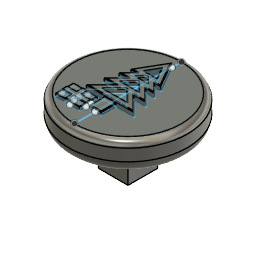
PIN6 (Autodesk Fusion 360 design; units mm, degrees)
Autodesk Fusion 360 part; units mm, degrees
sketch "Sketch1" plane through (0, 0, 0) normal (0, 1, 0) x (1, 0, 0)
  line L0 (0, 0) -> (5, 0)
  line L1 (5, 0) -> (5, 5)
  line L2 (5, 5) -> (0, 5)
  line L3 (0, 5) -> (0, 0)
  dimension "d1" = 5
  dimension "d2" = 5
  constraint horizontal L0
  constraint vertical L1
  constraint horizontal L2
  constraint vertical L3
  constraint coincident L0.start L3.end
  measures "d1" distance of L0.start L0.end
  measures "d2" distance of L0.start L2.end
extrude "Extrude1" add sketch "Sketch1" along normal blind 6
sketch "Sketch2" plane through (0, 6, 0) normal (0, 1, 0) x (-1, 0, 0)
  line L0 (0, -5) -> (0, 0)
  line L1 (0, 0) -> (-5, 0)
  line L2 (-5, 0) -> (-5, -5)
  line L3 (-5, -5) -> (0, -5)
  circle A0 centre (-2.5, -2.5) radius 10
  dimension "d5" = 20
  measures "d5" diameter of A0
extrude "Extrude2" add sketch "Sketch2" along normal blind 5 contours L0 L1 L2 L3 | A0
fillet "Fillet1" radius 2 1 edges at (11.8233, 6, -6.1162)
fillet "Fillet1" radius 1 1 edges at (11.8233, 11, -6.1162)
sketch "Sketch3" plane through (0, 11, 0) normal (0, 1, 0) x (-1, 0, 0)
  circle A0 centre (-2.5, -2.5) radius 9
  line L0 (-2.5, 6.5) -> (-2.5, -11.5)
  line L1 (-2.5, 3) -> (-3.5, 3)
  line L2 (-3.5, 3) -> (-3.5, 0.5)
  line L3 (-3.5, 0.5) -> (-6.5, 0.5)
  line L4 (-6.5, 0.5) -> (-4, -2)
  line L5 (-4, -2) -> (-6, -2)
  line L6 (-6, -2) -> (-4, -4)
  line L7 (-4, -4) -> (-5.5, -4)
  line L8 (-5.5, -4) -> (-4, -5.5)
  line L9 (-4, -5.5) -> (-5, -5.5)
  line L10 (-5, -5.5) -> (-2.5, -9.8301)
  line L11 (0.5, -4) -> (-1, -5.5)
  line L12 (-1, -2) -> (1, -2)
  line L13 (-1, -4) -> (0.5, -4)
  line L14 (-1.5, 0.5) -> (1.5, 0.5)
  line L15 (-2.5, 3) -> (-1.5, 3)
  line L16 (-1.5, 3) -> (-1.5, 0.5)
  line L17 (1.5, 0.5) -> (-1, -2)
  line L18 (0, -5.5) -> (-2.5, -9.8301)
  line L19 (1, -2) -> (-1, -4)
  line L20 (-1, -5.5) -> (0, -5.5)
  line L21 (-1.5, 0.5) -> (-3.5, 0.5)
  line L22 (-4.4238, -0.36) -> (-2.5, -2.2838)
  line L23 (-3.5, -0.36) -> (-4.4238, -0.36)
  line L24 (-1.5, -0.36) -> (-3.5, -0.36)
  line L25 (-1.5, -0.36) -> (-0.5762, -0.36)
  line L26 (-0.5762, -0.36) -> (-2.5, -2.2838)
  line L27 (-3.9238, -2.86) -> (-2.5, -4.2838)
  line L28 (-3.0762, -2.86) -> (-3.9238, -2.86)
  line L29 (-1.9238, -2.86) -> (-3.0762, -2.86)
  line L30 (-1.9238, -2.86) -> (-1.0762, -2.86)
  line L31 (-1.0762, -2.86) -> (-2.5, -4.2838)
  line L32 (-3.4238, -4.86) -> (-2.5, -5.7838)
  line L33 (-3.0762, -4.86) -> (-3.4238, -4.86)
  line L34 (-1.9238, -4.86) -> (-3.0762, -4.86)
  line L35 (-1.9238, -4.86) -> (-1.5762, -4.86)
  line L36 (-1.5762, -4.86) -> (-2.5, -5.7838)
  line L37 (-1.4896, -6.36) -> (-2.5, -8.1101)
  line L38 (-3.5104, -6.36) -> (-2.5, -8.1101)
  line L39 (-3.0762, -6.36) -> (-3.5104, -6.36)
  line L40 (-1.9238, -6.36) -> (-3.0762, -6.36)
  line L41 (-1.9238, -6.36) -> (-1.4896, -6.36)
  line L42 (3.0533, 1.123) -> (-0.9467, 1.123)
  line L43 (-0.9467, 1.123) -> (-0.9467, 4.123)
  line L44 (-0.9467, 4.123) -> (3.0533, 4.123)
  line L45 (3.0533, 4.123) -> (3.0533, 1.123)
  line L46 (1.4833, 4.123) -> (1.4833, 1.123)
  line L47 (1.0533, 4.123) -> (1.0533, 1.123)
  line L48 (1.0533, 2.623) -> (3.0533, 2.623)
  line L49 (3.0533, 2.193) -> (1.0533, 2.193)
  line L50 (3.0533, 3.053) -> (1.0533, 3.053)
  line L51 (0.6233, 4.123) -> (0.6233, 1.123)
  line L52 (-0.9467, 3.053) -> (1.0533, 3.053)
  line L53 (-0.9467, 2.193) -> (1.0533, 2.193)
  dimension "d12" = 60
  dimension "d19" = 0.86
  dimension "d28" = 4
  dimension "d29" = 3
  dimension "d30" = 0.43
  dimension "d31" = 0.43
  dimension "d36" = 2.5
  constraint coincident A0 L0.start
  constraint coincident A0 L0.end
  constraint vertical L0
  constraint coincident L0 L1.start
  constraint perpendicular L0 L1
  constraint perpendicular L1 L2
  constraint perpendicular L2 L3
  constraint perpendicular L2 L5
  constraint parallel L4 L6
  constraint parallel L4 L8
  constraint parallel L3 L9
  constraint coincident L0 L10.end
  constraint symmetric L0 L1.start L15.start
  constraint symmetric L0 L1.end L15.end
  constraint symmetric L0 L2.end L14.start
  constraint symmetric L0 L3.end L14.end
  constraint symmetric L0 L4.end L12.start
  constraint symmetric L0 L5.end L12.end
  constraint symmetric L0 L6.end L13.start
  constraint symmetric L0 L7.end L11.start
  constraint symmetric L0 L8.end L11.end
  constraint symmetric L0 L9.end L18.start
  constraint symmetric L0 L10.end L18.end
  constraint horizontal L42
  constraint vertical L43
  constraint horizontal L44
  constraint vertical L45
  constraint coincident L44 L46.start
  constraint coincident L42 L46.end
  constraint perpendicular L42 L46
  constraint midpoint L44 L47.start
  constraint midpoint L42 L47.end
  constraint midpoint L47 L48.start
  constraint midpoint L45 L48.end
  constraint coincident L45 L49.start
  constraint coincident L47 L49.end
  constraint perpendicular L47 L49
  constraint symmetric L48 L49.start L50.start
  constraint symmetric L48 L49.end L50.end
  constraint symmetric L46.start L47 L51.start
  constraint symmetric L46.end L47 L51.end
  constraint symmetric L47 L49.start L53.start
  constraint symmetric L47 L49.end L53.end
  constraint symmetric L47 L50.start L52.start
  constraint symmetric L47 L50.end L52.end
  measures "d12" angle of L9 L10
  measures "d28" distance of L42.start L42.end
  measures "d29" distance of L42.start L44.end
  measures "d30" distance of L46 L47
  measures "d31" distance of L48 L49
  measures "d36" distance of L1.end L2.end
extrude "Extrude5" add sketch "Sketch3" along normal blind 0.75 contours L0 L3 L4 L5 L6 L7 L8 L9 L10 L21 L22 L23 L24 L27 L28 L29 L32 L33 L34 L38 L39 L40 | L0 L11 L12 L13 L14 L17 L18 L19 L20 L21 L24 L25 L26 L29 L30 L31 L34 L35 L36 L37 L40 L41
extrude "Extrude6" add sketch "Sketch3" along normal blind 0.5 contours L0 L15 L16 L21 | L0 L1 L2 L21
fillet "Fillet2" radius 0.1 27 edges at (2.5, 11.75, -6.36) (3.0052, 11.75, -7.2351) (1.9948, 11.75, -7.2351) (1.25, 11.75, -7.6651) (0.5, 11.75, -5.5) (0.25, 11.75, -4.75) (0.25, 11.75, -4) (0, 11.75, -3) (0, 11.75, -2) (-0.25, 11.75, -0.75) (2.5, 11.75, 0.5) (5.25, 11.75, -0.75) (5, 11.75, -2) (5, 11.75, -3) (4.75, 11.75, -4) (4.75, 11.75, -4.75) (4.5, 11.75, -5.5) (3.75, 11.75, -7.6651) (2.9619, 11.75, -5.3219) (2.5, 11.75, -4.86) (2.0381, 11.75, -5.3219) (1.7881, 11.75, -3.5719) (3.2119, 11.75, -3.5719) (2.5, 11.75, -2.86) (3.4619, 11.75, -1.3219) (1.5381, 11.75, -1.3219) (2.5, 11.75, -0.36)
fillet "Fillet3" radius 0.1 3 edges at (1.5, 11.5, 1.75) (2.5, 11.5, 3) (3.5, 11.5, 1.75)
extrude "Extrude7" add sketch "Sketch3" along normal blind 0.5 contours L42 L45 L46 L49 | L42 L46 L47 L49 | L45 L46 L48 L49 | L42 L47 L51 L53 | L46 L47 L48 L49 | L45 L46 L48 L50 | L42 L43 L51 L53 | L47 L51 L52 L53 | L46 L47 L48 L50 | L44 L45 L46 L50 | L43 L51 L52 L53 | L44 L46 L47 L50 | L43 L44 L51 L52 | L44 L47 L51 L52
extrude "Extrude8" add sketch "Sketch3" along normal blind 0.6 contours L42 L46 L47 L49 | L45 L46 L48 L49 | L42 L47 L51 L53 | L46 L47 L48 L49 | L45 L46 L48 L50 | L47 L51 L52 L53 | L46 L47 L48 L50 | L43 L51 L52 L53 | L44 L46 L47 L50 | L44 L47 L51 L52
fillet "Fillet4" radius 0.05 12 edges at (-2.2683, 11.6, 3.053) (-3.0533, 11.6, 2.623) (-2.2683, 11.6, 2.193) (-1.4833, 11.6, 1.658) (-1.0533, 11.6, 1.123) (-0.6233, 11.6, 1.658) (0.1617, 11.6, 2.193) (0.9467, 11.6, 2.623) (0.1617, 11.6, 3.053) (-0.6233, 11.6, 3.588) (-1.0533, 11.6, 4.123) (-1.4833, 11.6, 3.588)
fillet "Fillet5" radius 0.05 8 edges at (-2.2683, 11.5, 4.123) (-3.0533, 11.5, 3.588) (-3.0533, 11.5, 1.658) (-2.2683, 11.5, 1.123) (0.1617, 11.5, 1.123) (0.9467, 11.5, 1.658) (0.9467, 11.5, 3.588) (0.1617, 11.5, 4.123)
extrude "Extrude3" [rolled back] along distance 0.5 taper angle 0
extrude "Extrude4" [rolled back] along distance 0.75 taper angle 0
